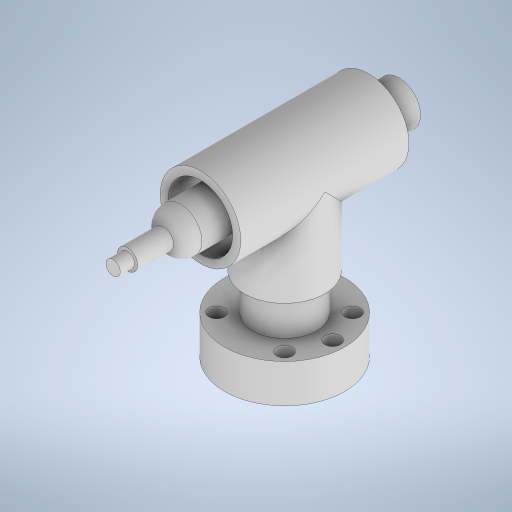
# Autodesk Inventor part: SoporteIRB
Saved by Autodesk Inventor 2023 (Build 270158000, 158)
## iProperties
Created: 2022-08-30
Part Number: SoporteIRB
Material: Generic
Document SubType Name: Modeling
Designer: andre
Density: 1 g/cm^3
Appearance: Default
Author: andre
Autodesk Inventor part; units mm, degrees
ref_plane "YZ Plane" through (0, 0, 0) normal (1, 0, 0) x (0, 1, 0)
ref_plane "XZ Plane" through (0, 0, 0) normal (0, 1, 0) x (-1, 0, 0)
ref_plane "XY Plane" through (0, 0, 0) normal (0, 0, 1) x (1, 0, 0)
sketch "Sketch1" plane through (0, 0, 0) normal (0, 0, 1) x (1, 0, 0)
  circle A0 centre (0, 0) radius 25
  dimension "d0" = 50
  constraints: 1 centre point, 1 coincident
  measures "d0" diameter of A0
extrude "Extrusion1" add sketch "Sketch1" along normal blind 16
sketch "Sketch2" plane through (0, 0, 16) normal (0, 0, 1) x (1, 0, 0)
  line L0 (0, 0) -> (-14.1421, 14.1421)
  line L1 (0, 0) -> (-17.9491, 0)
  point P0 (-14.1421, -14.1421)
  point P1 (-14.1421, -14.1421)
  point P2 (14.1421, -14.1421)
  point P3 (14.1421, -14.1421)
  point P4 (14.1421, 14.1421)
  point P5 (14.1421, 14.1421)
  point P6 (0, 20)
  dimension "d3" = 45
  dimension "d4" = 20
  dimension "d7" = 360
  dimension "d9" = 20
  constraints: 4 coincident, 4 end point, 1 horizontal, 9 other
  measures "d3" angle of L0 L1
  measures "d4" distance of L0.start L0.end
  measures "d9" distance from line of point (0, 20) L1
hole "Hole1" at (-14.1421, 14.1421, 16) at (-14.1421, -14.1421, 16) at (14.1421, -14.1421, 16) at (14.1421, 14.1421, 16) at (0, 20, 16) direction (0, 0, -1) diameter 6.5 end through all
sketch "Sketch3" plane through (0, 0, 16) normal (0, 0, 1) x (1, 0, 0)
  circle A0 centre (0, 0) radius 13.25
  dimension "d17" = 26.5
  constraints: 1 centre point, 1 coincident
  measures "d17" diameter of A0
extrude "Extrusion2" add sketch "Sketch3" along normal blind 15.1
sketch "Sketch4" plane through (0, 0, 31.1) normal (0, 0, 1) x (1, 0, 0)
  circle A0 centre (0, 0) radius 13.25 projected
  point P0 (13.25, 0)
  constraints: 1 horizontal alignment, 1 other
ref_plane "Work Plane1" through (13.25, 0, 31.1) normal (1, 0, 0) x (0, 1, 0)
sketch "Sketch5" plane through (13.25, 0, 31.1) normal (1, 0, 0) x (0, 1, 0)
  circle A0 centre (0, 36.75) radius 16.75
  line L0 (13.25, 0) -> (-13.25, 0) projected
  circle A1 centre (0, 36.75) radius 13.4
  point P0 (0, -31.1)
  dimension "d20" = 33.5
  dimension "d21" = 36.75
  dimension "d22" = 26.8
  constraints: 2 centre point, 1 coincident
  measures "d20" diameter of A0
  measures "d21" distance from line of A0.centre L0
  measures "d22" diameter of A1
extrude "Extrusion3" add sketch "Sketch5" along normal blind 21.75
sketch "Sketch6" plane through (13.25, 0, 67.85) normal (-1, 0, 0) x (0, 0, 1)
  circle A0 centre (0, 0) radius 16.75 projected
  circle A1 centre (0, 0) radius 13.4 projected
  point P0 (-67.85, 0)
extrude "Extrusion4" add sketch "Sketch6" along normal blind 13.25
sketch "Sketch7" plane through (0, 0, 67.85) normal (-1, 0, 0) x (0, 0, 1)
  circle A0 centre (0, 0) radius 16.75 projected
  circle A1 centre (0, 0) radius 13.4 projected
  point P0 (-67.85, 0)
extrude "Extrusion5" add sketch "Sketch7" along normal blind 35
sketch "Sketch8" plane through (0, 0, 31.1) normal (0, 0, 1) x (1, 0, 0)
  line L0 (35, -16.75) -> (35, 16.75) projected
  circle A0 centre (0, 0) radius 16.75
  dimension "d29" = 33.5
  constraints: 1 centre point, 1 coincident
  measures "d29" diameter of A0
extrude "Extrusion6" add sketch "Sketch8" along normal up to surface round surface about axis through (13.25, 0, 67.85) along (1, 0, 0) radius 16.75 far side no
sketch "Sketch9" plane through (-35, 0, 67.85) normal (-1, 0, 0) x (0, 0, 1)
  point P0 (-67.85, 0)
sketch "Sketch10" plane through (-35, 0, 67.85) normal (-1, 0, 0) x (0, 0, 1)
  circle A0 centre (0, 0) radius 16.75 projected
  point P0 (-67.85, 0)
  point P1 (0, 16.75)
  constraints: 1 coincident, 1 vertical alignment, 1 other
ref_plane "Work Plane3" through (-35, 0, 67.85) normal (0, 1, 0) x (-1, 0, 0)
ref_plane "Work Plane2" through (-35, 16.75, 67.85) normal (0, 1, 0) x (-1, 0, 0)
sketch "Sketch11" plane through (-35, 0, 67.85) normal (0, 1, 0) x (-1, 0, 0)
  line L0 (0, 0) -> (-70, 0)
  line L1 (-70, 0) -> (-70, 9)
  line L2 (-70, 9) -> (0, 9)
  line L3 (-88.4, 0) -> (-78.4, 0)
  line L4 (0, 0) -> (12.6, 0)
  line L5 (12.6, 0) -> (12.6, 9)
  line L6 (12.6, 9) -> (0, 9)
  line L7 (-88.4, 0) -> (-78.4, 0)
  line L8 (-70, -13.4) -> (-70, 13.4) construction
  line L9 (-70, 0) -> (-78.4, 0)
  line L10 (-78.4, 0) -> (-78.4, 9)
  line L11 (-78.4, 9) -> (-70, 9)
  line L12 (-70, 9) -> (-70, 0)
  line L13 (-78.4, 0) -> (-84.4, 0) construction
  line L14 (-84.4, 0) -> (-84.4, 4.25) construction
  line L15 (-78.4, 9) -> (-77.0307, 9) construction
  line L16 (-84.4, 0) -> (-84.4, 4.25) construction
  line L17 (-84.4, 4.25) -> (-85.3776, 4.25) construction
  line L18 (-4.2502, 6) -> (-4.2502, 22) construction
  line L19 (-4.2502, 22) -> (-3.0002, 22) construction
  line L20 (-100.4, 3) -> (-100.4, 0)
  line L21 (-3.0002, 22) -> (-3.0002, 28) construction
  line L22 (-3.0002, 28) -> (-0.0002, 28) construction
  line L23 (-106.4, 3) -> (-100.4, 3)
  arc A0 (-78.4, 9) -> (-85.3776, 4.25) centre (-78.4, 1.5) ccw
  line L24 (-85.3776, 4.25) -> (-100.4, 4.25)
  line L25 (-3.0002, 22) -> (-0.0002, 22) construction
  line L26 (-106.4, 0) -> (-106.4, 3)
  line L27 (-0.0002, 22) -> (-3.0002, 22) construction
  line L28 (-78.4, 9) -> (-78.4, 0)
  line L29 (-106.4, 0) -> (-78.4, 0)
  line L30 (-100.4, 0) -> (-100.4, 4.25)
  point P0 (-35, -67.85)
  point P1 (-88.4, 0)
  point P2 (-78.4, 0)
  point P3 (0, 9)
  point P4 (-70, 9)
  point P5 (-78.4, 9)
  dimension "d32" = 9
  dimension "d33" = 70
  dimension "d34" = 12.6
  dimension "d35" = 9
  dimension "d36" = 8.4
  dimension "d37" = 6
  dimension "d38" = 4.25
  dimension "d39" = 16
  dimension "d41" = 6
  dimension "d42" = 9
  constraints: 60 end point, 6 horizontal, 6 parallel, 6 perpendicular, 3 point on line, 2 point on circle, 1 centre point, 1 collinear
  measures "d32" distance between parallel lines of L2 L0
  measures "d33" distance of L2.end L1.end
  measures "d34" distance of L6.end L5.end
  measures "d35" distance of L9.end L10.end
  measures "d36" distance of L10.end L11.end
  measures "d37" distance of L13.start L13.end
  measures "d38" distance of L13.end L14.end
  measures "d39" distance of L14.end L24.end
  measures "d41" distance of L23.start L20.start
  measures "d42" distance from line of L9 L15.start
revolve "Revolution1" add sketch "Sketch11" angle 360 about axis through (71.4, 0, 67.85) along (-1, 0, 0)
equation "\"d35\" = d32"
equation "\"d42\" = d35"
body "Solid1"
